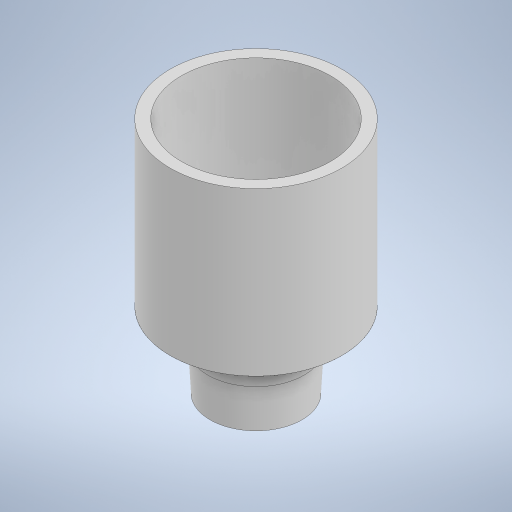
# Autodesk Inventor part: SoporteBombilla
Saved by Autodesk Inventor 2024 (Build 280153000, 153)
## iProperties
Created: 2023-12-01
Part Number: SoporteBombilla
Material: Genérico
Document SubType Name: Modeling
Designer: sergi
Density: 1 g/cm^3
Appearance: Valor por defecto
Author: sergi
Autodesk Inventor part; units mm, degrees
ref_plane "YZ Plane" through (0, 0, 0) normal (1, 0, 0) x (0, 1, 0)
ref_plane "XZ Plane" through (0, 0, 0) normal (0, 1, 0) x (-1, 0, 0)
ref_plane "XY Plane" through (0, 0, 0) normal (0, 0, 1) x (1, 0, 0)
sketch "Boceto1" plane through (0, 0, 0) normal (0, 1, 0) x (-1, 0, 0)
  circle A0 centre (0, 0) radius 19.7
  circle A1 centre (0, 0) radius 22.7
  dimension "d0" = 39.4
  dimension "d1" = 45.4
  constraints: 2 centre point, 2 coincident
  measures "d0" diameter of A0
  measures "d1" diameter of A1
extrude "Extrusión1" add sketch "Boceto1" along normal blind 40
sketch "Boceto2" plane through (0, 0, 0) normal (0, -1, 0) x (1, 0, 0)
  circle A0 centre (0, 0) radius 22.7 projected
  circle A1 centre (0, 0) radius 19.7 projected
extrude "Extrusión2" add sketch "Boceto2" along normal blind 3 contours A0 | A1
sketch "Boceto3" plane through (0, -3, 0) normal (0, -1, 0) x (1, 0, 0)
  circle A0 centre (0, 0) radius 10.2
  circle A1 centre (0, 0) radius 13.2
  dimension "d6" = 20.4
  dimension "d7" = 26.4
  constraints: 2 centre point, 2 coincident
  measures "d6" diameter of A0
  measures "d7" diameter of A1
extrude "Extrusión3" add sketch "Boceto3" along normal blind 20
chamfer "Chaflán1" distance 20 angle 3 1 edges at (-13.2, -23, 0) measured on face at (-13.2, -22.5, 0)
fillet "Empalme1" radius 10 2 edges at (-13.2, -3.0001, 0) (-13.2, -3, 0)
sketch "Boceto4" plane through (0, -3, 0) normal (0, -1, 0) x (1, 0, 0)
  circle A0 centre (0, 0) radius 10.2 projected
  constraints: 1 coincident
hole "Agujero1" at (0, -3, 0) direction (0, 1, 0) diameter 20.4 end through all
sketch "Boceto5" plane through (0, 0, 0) normal (1, 0, 0) x (0, 1, 0)
  line L0 (-23, -12.1518) -> (-23, 12.1518) projected
  line L1 (-12.4766, -12.7034) -> (-12.4766, 12.7034) projected
  line L2 (-12.4766, -12.7034) -> (-12.4766, 12.7034) projected
  line L3 (-3, 22.6896) -> (-3, -22.6896) projected
  line L4 (-23, -10.2) -> (-23, 10.2) projected
  line L5 (-23, 0) -> (-3, 0)
  line L6 (-3, 22.7) -> (-3, -22.7) projected
  line L7 (-23, 0) -> (-16.3333, 0)
  line L8 (-16.3333, 0) -> (-9.6667, 0)
  circle A0 centre (-16.3333, 0) radius 2.25
  circle A1 centre (-9.6667, 0) radius 2.25
  point P0 (0, 0)
  dimension "d21" = 6.6667
  dimension "d22" = 6.6667
  dimension "d23" = 4.5
  dimension "d24" = 4.5
  constraints: 6 end point, 2 centre point, 2 coincident, 2 midpoint, 2 point on line
  measures "d21" distance of L5.start L7.end
  measures "d22" distance of L7.end L8.end
  measures "d23" diameter of A0
  measures "d24" diameter of A1
hole "Agujero2" at (0, -16.3333, 0) at (0, -9.6667, 0) direction (-1, 0, 0) diameter 4.5 end through all
